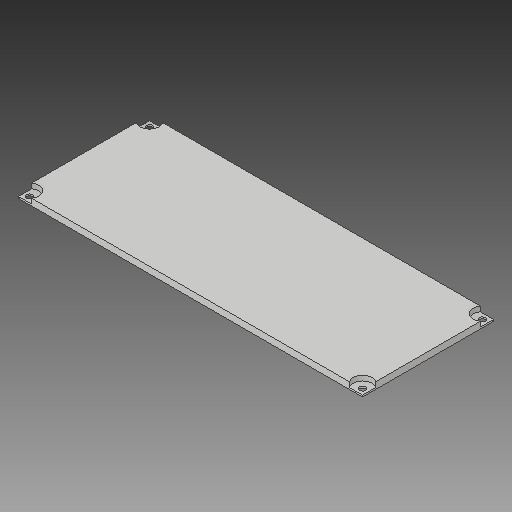
# Autodesk Inventor part: Access Panel
Saved by Autodesk Inventor 2018 (Build 220112000, 112)
## iProperties
Created: 2019-10-09
Part Number: Access Panel
Material: Generic
Document SubType Name: Modeling
Designer: Jacob
Density: 1 g/cm^3
Appearance: Default
Mass: 32.1065 g
Surface Area: 219.268 cm^2
Volume: 32.1065 cm^3
Author: Jacob
Autodesk Inventor part; units mm, degrees
ref_plane "YZ Plane" through (0, 0, 0) normal (1, 0, 0) x (0, 1, 0)
ref_plane "XZ Plane" through (0, 0, 0) normal (0, 1, 0) x (-1, 0, 0)
ref_plane "XY Plane" through (0, 0, 0) normal (0, 0, 1) x (1, 0, 0)
sketch "Sketch1" plane through (0, 0, 0) normal (0, 1, 0) x (-1, 0, 0)
  line L0 (82.55, -31.75) -> (-82.55, -31.75)
  line L1 (-82.55, -31.75) -> (-82.55, 31.75)
  line L2 (-82.55, 31.75) -> (82.55, 31.75)
  line L3 (82.55, 31.75) -> (82.55, -31.75)
  line L4 (82.55, -31.75) -> (-82.55, 31.75) construction
  line L5 (-82.55, -31.75) -> (82.55, 31.75) construction
  point P0 (0, 0)
  dimension "d0" = 165.1
  dimension "d1" = 63.5
  constraints: 12 end point, 2 midpoint, 2 parallel, 1 horizontal, 1 perpendicular
  measures "d0" distance of L0.start L0.end
  measures "d1" distance of L0.end L1.end
extrude "Extrusion1" add sketch "Sketch1" along normal blind 3.175
sketch "Sketch2" plane through (0, 3.175, 0) normal (0, 1, 0) x (1, 0, 0)
  line L0 (-76.2, 25.4) -> (76.2, 25.4) construction
  line L1 (76.2, 25.4) -> (76.2, -25.4) construction
  line L2 (76.2, -25.4) -> (-76.2, -25.4) construction
  line L3 (-76.2, -25.4) -> (-76.2, 25.4) construction
  line L4 (-76.2, 25.4) -> (76.2, -25.4) construction
  line L5 (76.2, 25.4) -> (-76.2, -25.4) construction
  line L6 (82.55, 31.75) -> (-82.55, 31.75) projected
  line L7 (82.55, -31.75) -> (82.55, 31.75) projected
  line L8 (-76.2, 0) -> (-82.55, 0) construction
  line L9 (-79.375, 0) -> (-79.375, -31.75) construction
  line L10 (-82.55, -31.75) -> (82.55, -31.75) projected
  line L11 (-79.375, 0) -> (-79.375, 31.75) construction
  line L12 (0, 25.4) -> (0, 31.75) construction
  line L13 (0, 28.575) -> (82.55, 28.575) construction
  line L14 (0, 28.575) -> (-82.55, 28.575) construction
  line L15 (0, -25.4) -> (0, -31.75) construction
  line L16 (0, -28.575) -> (-82.55, -28.575) construction
  line L17 (0, -28.575) -> (82.55, -28.575) construction
  line L18 (76.2, 0) -> (82.55, 0) construction
  line L19 (79.375, 0) -> (79.375, 31.75) construction
  line L20 (79.375, 0) -> (79.375, -31.75) construction
  circle A0 centre (-79.375, 28.575) radius 1.5
  circle A1 centre (-79.375, -28.575) radius 1.5
  circle A2 centre (79.375, -28.575) radius 1.5
  circle A3 centre (79.375, 28.575) radius 1.5
  point P0 (0, 0)
  dimension "d4" = 6.35
  dimension "d5" = 6.35
  dimension "d6" = 3
  dimension "d7" = 3
  dimension "d8" = 3
  dimension "d9" = 3
  constraints: 36 end point, 17 point on line, 13 midpoint, 5 perpendicular, 4 centre point, 2 horizontal, 2 parallel, 1 vertical
  measures "d4" distance between parallel lines of L6 L0
  measures "d5" distance between parallel lines of L7 L1
  measures "d6" diameter of A0
  measures "d7" diameter of A3
  measures "d8" diameter of A2
  measures "d9" diameter of A1
extrude "Extrusion2" cut sketch "Sketch2" against normal blind 3.175
sketch "Sketch3" plane through (0, 3.175, 0) normal (0, 1, 0) x (1, 0, 0)
  circle A0 centre (-79.375, 28.575) radius 1.5 projected
  circle A1 centre (-79.375, 28.575) radius 4.5
  circle A2 centre (-79.375, -28.575) radius 1.5 projected
  circle A3 centre (-79.375, -28.575) radius 4.5
  circle A4 centre (79.375, -28.575) radius 1.5 projected
  circle A5 centre (79.375, -28.575) radius 4.5
  circle A6 centre (79.375, 28.575) radius 1.5 projected
  circle A7 centre (79.375, 28.575) radius 4.5
  point P0 (0, 0)
  dimension "d12" = 9
  dimension "d13" = 9
  dimension "d14" = 9
  dimension "d15" = 9
  constraints: 4 centre point, 4 coincident
  measures "d12" diameter of A7
  measures "d13" diameter of A5
  measures "d14" diameter of A3
  measures "d15" diameter of A1
extrude "Extrusion3" cut sketch "Sketch3" against normal blind 2.3813
sketch "Sketch4" plane through (0, 3.175, 0) normal (0, 1, 0) x (1, 0, 0)
  line L0 (82.55, -31.75) -> (-82.55, -31.75) projected
  line L1 (82.55, 31.75) -> (82.55, 25.3861) projected
  line L2 (-82.55, -31.75) -> (82.55, -31.75)
  line L3 (82.55, -31.75) -> (82.55, 31.75)
  line L4 (82.55, 31.75) -> (-82.55, 31.75)
  line L5 (-82.55, 31.75) -> (-82.55, -31.75)
  line L6 (-82.05, -31.25) -> (82.05, -31.25)
  line L7 (82.05, -31.25) -> (82.05, 31.25)
  line L8 (82.05, 31.25) -> (-82.05, 31.25)
  line L9 (-82.05, 31.25) -> (-82.05, -31.25)
  line L10 (-82.05, -31.25) -> (82.05, 31.25) construction
  line L11 (82.05, -31.25) -> (-82.05, 31.25) construction
  point P0 (0, 0)
  dimension "d18" = 0.5
  dimension "d19" = 0.5
  constraints: 20 end point, 4 parallel, 2 horizontal, 2 midpoint, 2 perpendicular
  measures "d18" distance between parallel lines of L5 L9
  measures "d19" distance between parallel lines of L0 L6
extrude "Extrusion4" cut sketch "Sketch4" against normal blind 25.4
body "Solid1"
